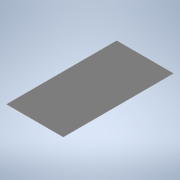
# Autodesk Inventor part: priklop
Saved by Autodesk Inventor 2022 (Build 260153000, 153)
## iProperties
Created: 2022-12-16
Part Number: priklop
Material: Generic
Document SubType Name: Modeling
Designer: matys
Density: 1 g/cm^3
Appearance: Gray
Author: matys
Autodesk Inventor part; units mm, degrees
ref_plane "YZ Plane" through (0, 0, 0) normal (1, 0, 0) x (0, 1, 0)
ref_plane "XZ Plane" through (0, 0, 0) normal (0, 1, 0) x (-1, 0, 0)
ref_plane "XY Plane" through (0, 0, 0) normal (0, 0, 1) x (1, 0, 0)
sketch "Sketch1" plane through (0, 0, 0) normal (0, 1, 0) x (-1, 0, 0)
  line L0 (0, 0) -> (0, -110)
  line L1 (0, -110) -> (56.8, -110)
  line L2 (56.8, -110) -> (56.8, 0)
  line L3 (56.8, 0) -> (0, 0)
  dimension "d0" = 110
  dimension "d1" = 56.8
  constraints: 8 end point, 2 perpendicular, 1 horizontal, 1 vertical
  measures "d0" distance of L0.start L0.end
  measures "d1" distance of L0.end L1.end
extrude "Extrusion1" add sketch "Sketch1" along normal blind 2
chamfer "Chamfer1" distance 2 angle 45 1 edges at (0, 0, -55)
chamfer "Chamfer2" distance 2 angle 45 1 edges at (-56.8, 0, -55)
chamfer "Chamfer3" distance 2 angle 45 2 edges at (-28.4, 0, 0) (-28.4, 0, -110)
body "Solid1"
